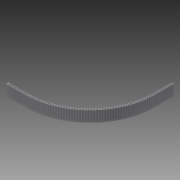
# Autodesk Inventor part: Runner Rails 6 v1
Saved by Autodesk Inventor 2013 (Build 170138000, 138)
## iProperties
Created: 2013-01-16
Part Number: Runner Rails 6 v1
Material: Polycarbonate, Clear
Document SubType Name: Modeling
Designer: actoennies
Mass: 344.82 g
Surface Area: 1847.27 cm^2
Volume: 385.704 cm^3
Density: 0.894 g/cm^3
Author: actoennies
Autodesk Inventor part; units mm, degrees
ref_plane "YZ Plane" through (0, 0, 0) normal (1, 0, 0) x (0, 1, 0)
ref_plane "XZ Plane" through (0, 0, 0) normal (0, 1, 0) x (-1, 0, 0)
ref_plane "XY Plane" through (0, 0, 0) normal (0, 0, 1) x (1, 0, 0)
sketch "Sketch1" plane through (0, 0, 0) normal (0, 1, 0) x (-1, 0, 0)
  circle A0 centre (-336.55, 0) radius 3.3782
  circle A1 centre (-234.3065, 241.5985) radius 3.3782
  circle A2 centre (-241.5985, 234.3065) radius 3.3782
  circle A3 centre (87.8158, 336.55) radius 3.3782
  circle A4 centre (0, 336.55) radius 3.3782
  arc A5 (0, 342.9) -> (-342.9, 0) centre (0, 0) ccw
  arc A6 (0, 330.2) -> (-330.2, 0) centre (0, 0) ccw
  line L0 (-342.9, 0) -> (-342.9, -101.6)
  line L1 (-342.9, -101.6) -> (-330.2, -101.6)
  line L2 (-330.2, -101.6) -> (-330.2, 0)
  circle A7 centre (-336.55, -9.525) radius 3.3782
  circle A8 centre (-336.55, -19.05) radius 3.3782
  circle A9 centre (-336.55, -28.575) radius 3.3782
  circle A10 centre (-336.55, -38.1) radius 3.3782
  circle A11 centre (-336.55, -47.625) radius 3.3782
  circle A12 centre (-336.55, -57.15) radius 3.3782
  circle A13 centre (-336.55, -66.675) radius 3.3782
  circle A14 centre (-336.55, -76.2) radius 3.3782
  circle A15 centre (-336.55, -85.725) radius 3.3782
  circle A16 centre (-336.55, -95.25) radius 3.3782
  line L3 (0, 330.2) -> (101.6, 330.2)
  line L4 (101.6, 330.2) -> (101.6, 342.9)
  line L5 (101.6, 342.9) -> (0, 342.9)
  circle A17 centre (-10.3511, 336.3908) radius 3.3782
  circle A18 centre (-20.6925, 335.9133) radius 3.3782
  circle A19 centre (-31.0142, 335.1179) radius 3.3782
  circle A20 centre (-41.3066, 334.0055) radius 3.3782
  circle A21 centre (-51.5599, 332.577) radius 3.3782
  circle A22 centre (-61.7645, 330.8339) radius 3.3782
  circle A23 centre (-71.9106, 328.7777) radius 3.3782
  circle A24 centre (-81.9886, 326.4104) radius 3.3782
  circle A25 centre (-91.9891, 323.7343) radius 3.3782
  circle A26 centre (-101.9026, 320.7519) radius 3.3782
  circle A27 centre (-111.7196, 317.466) radius 3.3782
  circle A28 centre (-121.4309, 313.8797) radius 3.3782
  circle A29 centre (-131.0273, 309.9964) radius 3.3782
  circle A30 centre (-140.4997, 305.8198) radius 3.3782
  circle A31 centre (-149.8392, 301.3538) radius 3.3782
  circle A32 centre (-159.037, 296.6027) radius 3.3782
  circle A33 centre (-168.0842, 291.5709) radius 3.3782
  circle A34 centre (-176.9724, 286.2633) radius 3.3782
  circle A35 centre (-185.6932, 280.6848) radius 3.3782
  circle A36 centre (-194.2382, 274.8407) radius 3.3782
  circle A37 centre (-202.5995, 268.7366) radius 3.3782
  circle A38 centre (-210.769, 262.3782) radius 3.3782
  circle A39 centre (-218.7392, 255.7715) radius 3.3782
  circle A40 centre (-226.5024, 248.9228) radius 3.3782
  circle A41 centre (-336.3908, 10.3511) radius 3.3782
  circle A42 centre (-335.9133, 20.6925) radius 3.3782
  circle A43 centre (-335.1179, 31.0142) radius 3.3782
  circle A44 centre (-334.0055, 41.3066) radius 3.3782
  circle A45 centre (-332.577, 51.5599) radius 3.3782
  circle A46 centre (-330.8339, 61.7645) radius 3.3782
  circle A47 centre (-328.7777, 71.9106) radius 3.3782
  circle A48 centre (-326.4104, 81.9886) radius 3.3782
  circle A49 centre (-323.7343, 91.9891) radius 3.3782
  circle A50 centre (-320.7519, 101.9026) radius 3.3782
  circle A51 centre (-317.466, 111.7196) radius 3.3782
  circle A52 centre (-313.8797, 121.4309) radius 3.3782
  circle A53 centre (-309.9964, 131.0273) radius 3.3782
  circle A54 centre (-305.8198, 140.4997) radius 3.3782
  circle A55 centre (-301.3538, 149.8392) radius 3.3782
  circle A56 centre (-296.6027, 159.037) radius 3.3782
  circle A57 centre (-291.5709, 168.0842) radius 3.3782
  circle A58 centre (-286.2633, 176.9724) radius 3.3782
  circle A59 centre (-280.6848, 185.6932) radius 3.3782
  circle A60 centre (-274.8407, 194.2382) radius 3.3782
  circle A61 centre (-268.7366, 202.5995) radius 3.3782
  circle A62 centre (-262.3782, 210.769) radius 3.3782
  circle A63 centre (-255.7715, 218.7392) radius 3.3782
  circle A64 centre (-248.9228, 226.5024) radius 3.3782
  circle A65 centre (9.525, 336.55) radius 3.3782
  circle A66 centre (19.05, 336.55) radius 3.3782
  circle A67 centre (28.575, 336.55) radius 3.3782
  circle A68 centre (38.1, 336.55) radius 3.3782
  circle A69 centre (47.625, 336.55) radius 3.3782
  circle A70 centre (57.15, 336.55) radius 3.3782
  circle A71 centre (66.675, 336.55) radius 3.3782
  circle A72 centre (76.2, 336.55) radius 3.3782
  line L6 (0, 325.5916) -> (0, 330.2)
  line L7 (0, 342.9) -> (0, 348.9307)
  dimension "d2" = 101.6
  dimension "d5" = 9.525
  dimension "d10" = 101.6
  dimension "d13" = 42.3
  dimension "d17" = 42.3
  dimension "d21" = 9.525
  constraints: 73 centre point, 16 end point, 4 parallel, 4 perpendicular, 4 point on circle, 4 tangent, 1 coincident, 1 horizontal, 1 vertical, 134 other
  measures "d2" distance of L0.start L0.end
  measures "d5" distance of A0.centre A7.centre
  measures "d10" distance of L5.end L4.end
  measures "d21" distance of A4.centre A65.centre
extrude "Extrusion1" add sketch "Sketch1" along normal blind 57.15
body "Solid1"
